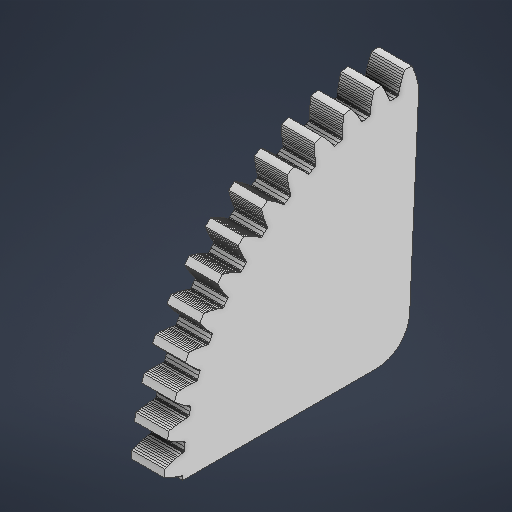
# Autodesk Inventor part: pitch gear v3
Saved by Autodesk Inventor 2026.2 (Build 302298000, 298)
## iProperties
Created: 2026-01-17
Part Number: pitch gear v3
Material: Generic
Document SubType Name: Modeling
Designer: User
Density: 1 g/cm^3
Appearance: Default
Author: User
Autodesk Inventor part; units mm, degrees
(part 1 of 2)
ref_plane "YZ Plane" through (0, 0, 0) normal (1, 0, 0) x (0, 1, 0)
ref_plane "XZ Plane" through (0, 0, 0) normal (0, 1, 0) x (-1, 0, 0)
ref_plane "XY Plane" through (0, 0, 0) normal (0, 0, 1) x (1, 0, 0)
sketch "Sketch1" plane through (0, 0, 0) normal (1, 0, 0) x (0, 1, 0)
  line L0 (51.3338, 5.5368) -> (50.9543, 5.3173)
  line L1 (50.9543, 5.3173) -> (50.5888, 5.1158)
  line L2 (50.5888, 5.1158) -> (50.2381, 4.9321)
  line L3 (50.2381, 4.9321) -> (49.9008, 4.7642)
  line L4 (49.9008, 4.7642) -> (49.5784, 4.6121)
  line L5 (49.5784, 4.6121) -> (49.2732, 4.4759)
  line L6 (49.2732, 4.4759) -> (48.9827, 4.3535)
  line L7 (48.9827, 4.3535) -> (48.455, 4.15)
  line L8 (48.455, 4.15) -> (48.0445, 4.0082)
  line L9 (48.0445, 4.0082) -> (47.95, 3.9663)
  line L10 (47.95, 3.9663) -> (47.8784, 3.9226)
  line L11 (47.8784, 3.9226) -> (47.8295, 3.8782)
  line L12 (47.8295, 3.8782) -> (47.8036, 3.8338)
  line L13 (47.8036, 3.8338) -> (47.7992, 3.812)
  line L14 (47.7992, 3.812) -> (47.812, 3.6369)
  line L15 (47.812, 3.6369) -> (47.8554, 3.0108)
  line L16 (47.8554, 3.0108) -> (47.8909, 2.3842)
  line L17 (47.8909, 2.3842) -> (47.9, 2.2089)
  line L18 (47.9, 2.2089) -> (47.9072, 2.1878)
  line L19 (47.9072, 2.1878) -> (47.9385, 2.1471)
  line L20 (47.9385, 2.1471) -> (47.9925, 2.1091)
  line L21 (47.9925, 2.1091) -> (48.069, 2.0748)
  line L22 (48.069, 2.0748) -> (48.168, 2.045)
  line L23 (48.168, 2.045) -> (48.593, 1.9557)
  line L24 (48.593, 1.9557) -> (49.1421, 1.82)
  line L25 (49.1421, 1.82) -> (49.4456, 1.735)
  line L26 (49.4456, 1.735) -> (49.7655, 1.6381)
  line L27 (49.7655, 1.6381) -> (50.1044, 1.5276)
  line L28 (50.1044, 1.5276) -> (50.4601, 1.4033)
  line L29 (50.4601, 1.4033) -> (50.8311, 1.265)
  line L30 (50.8311, 1.265) -> (51.219, 1.1109)
  line L31 (51.219, 1.1109) -> (51.623, 0.9407)
  line L32 (51.623, 0.9407) -> (51.9942, 0.7753)
  arc A0 (51.9942, -0.7753) -> (51.9942, 0.7753) centre (0, 0) ccw
  line L33 (51.9942, -0.7753) -> (51.623, -0.9407)
  line L34 (51.623, -0.9407) -> (51.219, -1.1109)
  line L35 (51.219, -1.1109) -> (50.8311, -1.265)
  line L36 (50.8311, -1.265) -> (50.4601, -1.4033)
  line L37 (50.4601, -1.4033) -> (50.1044, -1.5276)
  line L38 (50.1044, -1.5276) -> (49.7655, -1.6381)
  line L39 (49.7655, -1.6381) -> (49.4456, -1.735)
  line L40 (49.4456, -1.735) -> (49.1421, -1.82)
  line L41 (49.1421, -1.82) -> (48.593, -1.9557)
  line L42 (48.593, -1.9557) -> (48.168, -2.045)
  line L43 (48.168, -2.045) -> (48.069, -2.0748)
  line L44 (48.069, -2.0748) -> (47.9925, -2.1091)
  line L45 (47.9925, -2.1091) -> (47.9385, -2.1471)
  line L46 (47.9385, -2.1471) -> (47.9072, -2.1878)
  line L47 (47.9072, -2.1878) -> (47.9, -2.2089)
  line L48 (47.9, -2.2089) -> (47.8961, -2.2835)
  line L49 (0, 47.95) -> (0.6276, 47.9461)
  line L50 (0.6276, 47.9461) -> (0.8032, 47.9442)
  line L51 (0.8032, 47.9442) -> (0.8247, 47.95)
  line L52 (0.8247, 47.95) -> (0.8673, 47.9787)
  line L53 (0.8673, 47.9787) -> (0.9086, 48.0302)
  line L54 (0.9086, 48.0302) -> (0.9476, 48.1044)
  line L55 (0.9476, 48.1044) -> (0.9835, 48.2014)
  line L56 (0.9835, 48.2014) -> (1.0993, 48.6199)
  line L57 (1.0993, 48.6199) -> (1.2692, 49.1594)
  line L58 (1.2692, 49.1594) -> (1.3732, 49.457)
  line L59 (1.3732, 49.457) -> (1.49, 49.7701)
  line L60 (1.49, 49.7701) -> (1.6215, 50.1014)
  line L61 (1.6215, 50.1014) -> (1.7678, 50.4486)
  line L62 (1.7678, 50.4486) -> (1.9293, 50.8102)
  line L63 (1.9293, 50.8102) -> (2.1073, 51.1877)
  line L64 (2.1073, 51.1877) -> (2.3026, 51.5802)
  line L65 (2.3026, 51.5802) -> (2.4909, 51.9403)
  arc A1 (4.0386, 51.8429) -> (2.4909, 51.9403) centre (0, 0) ccw
  line L66 (4.0386, 51.8429) -> (4.1802, 51.4621)
  line L67 (4.1802, 51.4621) -> (4.3248, 51.0482)
  line L68 (4.3248, 51.0482) -> (4.4542, 50.6514)
  line L69 (4.4542, 50.6514) -> (4.569, 50.2724)
  line L70 (4.569, 50.2724) -> (4.6707, 49.9096)
  line L71 (4.6707, 49.9096) -> (4.7596, 49.5644)
  line L72 (4.7596, 49.5644) -> (4.8363, 49.2391)
  line L73 (4.8363, 49.2391) -> (4.9021, 48.9308)
  line L74 (4.9021, 48.9308) -> (5.003, 48.3743)
  line L75 (5.003, 48.3743) -> (5.0655, 47.9445)
  line L76 (5.0655, 47.9445) -> (5.0889, 47.8439)
  line L77 (5.0889, 47.8439) -> (5.1184, 47.7653)
  line L78 (5.1184, 47.7653) -> (5.1529, 47.7091)
  line L79 (5.1529, 47.7091) -> (5.1916, 47.6753)
  line L80 (5.1916, 47.6753) -> (5.2122, 47.6668)
  line L81 (5.2122, 47.6668) -> (5.3866, 47.6467)
  line L82 (5.3866, 47.6467) -> (6.0097, 47.5719)
  line L83 (6.0097, 47.5719) -> (6.6319, 47.4893)
  line L84 (6.6319, 47.4893) -> (6.8058, 47.4655)
  line L85 (6.8058, 47.4655) -> (6.8279, 47.4685)
  line L86 (6.8279, 47.4685) -> (6.8737, 47.4917)
  line L87 (6.8737, 47.4917) -> (6.9212, 47.5376)
  line L88 (6.9212, 47.5376) -> (6.9692, 47.6063)
  line L89 (6.9692, 47.6063) -> (7.017, 47.698)
  line L90 (7.017, 47.698) -> (7.1844, 48.0988)
  line L91 (7.1844, 48.0988) -> (7.4205, 48.6127)
  line L92 (7.4205, 48.6127) -> (7.5609, 48.8949)
  line L93 (7.5609, 48.8949) -> (7.7161, 49.1909)
  line L94 (7.7161, 49.1909) -> (7.8881, 49.5031)
  line L95 (7.8881, 49.5031) -> (8.0768, 49.8293)
  line L96 (8.0768, 49.8293) -> (8.2822, 50.1678)
  line L97 (8.2822, 50.1678) -> (8.5062, 50.5199)
  line L98 (8.5062, 50.5199) -> (8.7492, 50.8849)
  line L99 (8.7492, 50.8849) -> (8.9811, 51.2185)
  arc A2 (10.5044, 50.928) -> (8.9811, 51.2185) centre (0, 0) ccw
  line L100 (10.5044, 50.928) -> (10.5972, 50.5323)
  line L101 (10.5972, 50.5323) -> (10.6888, 50.1036)
  line L102 (10.6888, 50.1036) -> (10.7673, 49.6937)
  line L103 (10.7673, 49.6937) -> (10.8338, 49.3033)
  line L104 (10.8338, 49.3033) -> (10.8892, 48.9306)
  line L105 (10.8892, 48.9306) -> (10.9342, 48.5771)
  line L106 (10.9342, 48.5771) -> (10.9694, 48.2447)
  line L107 (10.9694, 48.2447) -> (10.9961, 47.9306)
  line L108 (10.9961, 47.9306) -> (11.0265, 47.3658)
  line L109 (11.0265, 47.3658) -> (11.0346, 46.9316)
  line L110 (11.0346, 46.9316) -> (11.0452, 46.8288)
  line L111 (11.0452, 46.8288) -> (11.0646, 46.7472)
  line L112 (11.0646, 46.7472) -> (11.0918, 46.687)
  line L113 (11.0918, 46.687) -> (11.1259, 46.6486)
  line L114 (11.1259, 46.6486) -> (11.1453, 46.6377)
  line L115 (11.1453, 46.6377) -> (11.3158, 46.5958)
  line L116 (11.3158, 46.5958) -> (11.9247, 46.4436)
  line L117 (11.9247, 46.4436) -> (12.5316, 46.2837)
  line L118 (12.5316, 46.2837) -> (12.7012, 46.2382)
  line L119 (12.7012, 46.2382) -> (12.7234, 46.2385)
  line L120 (12.7234, 46.2385) -> (12.7718, 46.2557)
  line L121 (12.7718, 46.2557) -> (12.8246, 46.2953)
  line L122 (12.8246, 46.2953) -> (12.8809, 46.3575)
  line L123 (12.8809, 46.3575) -> (12.9398, 46.4424)
  line L124 (12.9398, 46.4424) -> (13.1561, 46.819)
  line L125 (13.1561, 46.819) -> (13.4548, 47.2993)
  line L126 (13.4548, 47.2993) -> (13.6295, 47.5617)
  line L127 (13.6295, 47.5617) -> (13.8205, 47.836)
  line L128 (13.8205, 47.836) -> (14.0303, 48.1242)
  line L129 (14.0303, 48.1242) -> (14.2584, 48.4241)
  line L130 (14.2584, 48.4241) -> (14.5046, 48.7341)
  line L131 (14.5046, 48.7341) -> (14.771, 49.0554)
  line L132 (14.771, 49.0554) -> (15.0578, 49.3871)
  line L133 (15.0578, 49.3871) -> (15.3297, 49.689)
  arc A3 (16.8045, 49.2098) -> (15.3297, 49.689) centre (0, 0) ccw
  line L134 (16.8045, 49.2098) -> (16.847, 48.8057)
  line L135 (16.847, 48.8057) -> (16.8841, 48.3688)
  line L136 (16.8841, 48.3688) -> (16.9107, 47.9523)
  line L137 (16.9107, 47.9523) -> (16.9277, 47.5567)
  line L138 (16.9277, 47.5567) -> (16.9359, 47.18)
  line L139 (16.9359, 47.18) -> (16.9363, 46.8236)
  line L140 (16.9363, 46.8236) -> (16.9296, 46.4894)
  line L141 (16.9296, 46.4894) -> (16.9167, 46.1745)
  line L142 (16.9167, 46.1745) -> (16.876, 45.6104)
  line L143 (16.876, 45.6104) -> (16.8297, 45.1785)
  line L144 (16.8297, 45.1785) -> (16.8273, 45.0752)
  line L145 (16.8273, 45.0752) -> (16.8363, 44.9918)
  line L146 (16.8363, 44.9918) -> (16.8558, 44.9287)
  line L147 (16.8558, 44.9287) -> (16.8848, 44.8864)
  line L148 (16.8848, 44.8864) -> (16.9027, 44.8731)
  line L149 (16.9027, 44.8731) -> (17.0666, 44.8102)
  line L150 (17.0666, 44.8102) -> (17.6516, 44.5828)
  line L151 (17.6516, 44.5828) -> (18.2337, 44.3481)
  line L152 (18.2337, 44.3481) -> (18.3962, 44.2817)
  line L153 (18.3962, 44.2817) -> (18.4183, 44.2792)
  line L154 (18.4183, 44.2792) -> (18.4685, 44.2902)
  line L155 (18.4685, 44.2902) -> (18.5258, 44.3229)
  line L156 (18.5258, 44.3229) -> (18.5895, 44.3775)
  line L157 (18.5895, 44.3775) -> (18.6585, 44.4544)
  line L158 (18.6585, 44.4544) -> (18.9203, 44.801)
  line L159 (18.9203, 44.801) -> (19.2769, 45.24)
  line L160 (19.2769, 45.24) -> (19.4831, 45.4785)
  line L161 (19.4831, 45.4785) -> (19.7069, 45.7266)
  line L162 (19.7069, 45.7266) -> (19.9512, 45.9862)
  line L163 (19.9512, 45.9862) -> (20.2151, 46.2552)
  line L164 (20.2151, 46.2552) -> (20.4983, 46.5319)
  line L165 (20.4983, 46.5319) -> (20.8028, 46.8173)
  line L166 (20.8028, 46.8173) -> (21.1289, 47.1104)
  line L167 (21.1289, 47.1104) -> (21.4365, 47.3759)
  arc A4 (22.8396, 46.7156) -> (21.4365, 47.3759) centre (0, 0) ccw
  line L168 (22.8396, 46.7156) -> (22.8311, 46.3094)
  line L169 (22.8311, 46.3094) -> (22.8132, 45.8713)
  line L170 (22.8132, 45.8713) -> (22.7874, 45.4547)
  line L171 (22.7874, 45.4547) -> (22.7546, 45.0601)
  line L172 (22.7546, 45.0601) -> (22.7156, 44.6854)
  line L173 (22.7156, 44.6854) -> (22.6713, 44.3317)
  line L174 (22.6713, 44.3317) -> (22.6228, 44.001)
  line L175 (22.6228, 44.001) -> (22.5705, 43.6902)
  line L176 (22.5705, 43.6902) -> (22.4595, 43.1356)
  line L177 (22.4595, 43.1356) -> (22.3593, 42.713)
  line L178 (22.3593, 42.713) -> (22.3441, 42.6107)
  line L179 (22.3441, 42.6107) -> (22.3425, 42.5269)
  line L180 (22.3425, 42.5269) -> (22.3539, 42.4618)
  line L181 (22.3539, 42.4618) -> (22.3774, 42.4162)
  line L182 (22.3774, 42.4162) -> (22.3935, 42.4008)
  line L183 (22.3935, 42.4008) -> (22.5482, 42.3178)
  line L184 (22.5482, 42.3178) -> (23.1001, 42.0189)
  line L185 (23.1001, 42.0189) -> (23.6482, 41.7131)
  line L186 (23.6482, 41.7131) -> (23.8011, 41.6269)
  line L187 (23.8011, 41.6269) -> (23.8227, 41.6216)
  line L188 (23.8227, 41.6216) -> (23.8739, 41.6262)
  line L189 (23.8739, 41.6262) -> (23.9349, 41.6515)
  line L190 (23.9349, 41.6515) -> (24.0049, 41.6977)
  line L191 (24.0049, 41.6977) -> (24.083, 41.7654)
  line L192 (24.083, 41.7654) -> (24.3862, 42.0763)
  line L193 (24.3862, 42.0763) -> (24.7949, 42.4673)
  line L194 (24.7949, 42.4673) -> (25.0294, 42.678)
  line L195 (25.0294, 42.678) -> (25.2826, 42.8961)
  line L196 (25.2826, 42.8961) -> (25.5575, 43.1231)
  line L197 (25.5575, 43.1231) -> (25.853, 43.3568)
  line L198 (25.853, 43.3568) -> (26.1686, 43.5959)
  line L199 (26.1686, 43.5959) -> (26.5065, 43.8409)
  line L200 (26.5065, 43.8409) -> (26.8668, 44.0908)
  line L201 (26.8668, 44.0908) -> (27.2052, 44.3156)
  arc A5 (28.5145, 43.4847) -> (27.2052, 44.3156) centre (0, 0) ccw
  line L202 (28.5145, 43.4847) -> (28.4552, 43.0827)
  line L203 (28.4552, 43.0827) -> (28.3825, 42.6503)
  line L204 (28.3825, 42.6503) -> (28.3047, 42.2403)
  line L205 (28.3047, 42.2403) -> (28.2227, 41.8529)
  line L206 (28.2227, 41.8529) -> (28.1371, 41.486)
  line L207 (28.1371, 41.486) -> (28.0488, 41.1407)
  line L208 (28.0488, 41.1407) -> (27.9592, 40.8187)
  line L209 (27.9592, 40.8187) -> (27.8684, 40.5168)
  line L210 (27.8684, 40.5168) -> (27.6887, 39.9805)
  line L211 (27.6887, 39.9805) -> (27.5364, 39.5738)
  line L212 (27.5364, 39.5738) -> (27.5084, 39.4743)
  line L213 (27.5084, 39.4743) -> (27.4964, 39.3913)
  line L214 (27.4964, 39.3913) -> (27.4995, 39.3253)
  line L215 (27.4995, 39.3253) -> (27.5171, 39.2771)
  line L216 (27.5171, 39.2771) -> (27.5311, 39.2598)
  line L217 (27.5311, 39.2598) -> (27.6742, 39.1581)
  line L218 (27.6742, 39.1581) -> (28.1843, 38.7924)
  line L219 (28.1843, 38.7924) -> (28.6898, 38.4203)
  line L220 (28.6898, 38.4203) -> (28.8307, 38.3156)
  line L221 (28.8307, 38.3156) -> (28.8515, 38.3076)
  line L222 (28.8515, 38.3076) -> (28.9028, 38.3058)
  line L223 (28.9028, 38.3058) -> (28.9665, 38.3232)
  line L224 (28.9665, 38.3232) -> (29.0417, 38.3603)
  line L225 (29.0417, 38.3603) -> (29.1277, 38.4176)
  line L226 (29.1277, 38.4176) -> (29.4675, 38.6882)
  line L227 (29.4675, 38.6882) -> (29.922, 39.0248)
  line L228 (29.922, 39.0248) -> (30.181, 39.2044)
  line L229 (30.181, 39.2044) -> (30.4596, 39.3891)
  line L230 (30.4596, 39.3891) -> (30.7607, 39.5798)
  line L231 (30.7607, 39.5798) -> (31.0832, 39.7747)
  line L232 (31.0832, 39.7747) -> (31.4263, 39.9723)
  line L233 (31.4263, 39.9723) -> (31.7922, 40.173)
  line L234 (31.7922, 40.173) -> (32.1809, 40.3758)
  line L235 (32.1809, 40.3758) -> (32.5449, 40.5565)
  arc A6 (33.7398, 39.568) -> (32.5449, 40.5565) centre (0, 0) ccw
  line L236 (33.7398, 39.568) -> (33.6305, 39.1766)
  line L237 (33.6305, 39.1766) -> (33.5042, 38.7568)
  line L238 (33.5042, 38.7568) -> (33.3756, 38.3597)
  line L239 (33.3756, 38.3597) -> (33.2458, 37.9857)
  line L240 (33.2458, 37.9857) -> (33.1148, 37.6324)
  line L241 (33.1148, 37.6324) -> (32.9839, 37.3008)
  line L242 (32.9839, 37.3008) -> (32.8546, 36.9926)
  line L243 (32.8546, 36.9926) -> (32.7267, 36.7045)
  line L244 (32.7267, 36.7045) -> (32.4812, 36.1949)
  line L245 (32.4812, 36.1949) -> (32.2791, 35.8105)
  line L246 (32.2791, 35.8105) -> (32.239, 35.7153)
  line L247 (32.239, 35.7153) -> (32.2166, 35.6344)
  line L248 (32.2166, 35.6344) -> (32.2115, 35.5686)
  line L249 (32.2115, 35.5686) -> (32.2229, 35.5186)
  line L250 (32.2229, 35.5186) -> (32.2346, 35.4996)
  line L251 (32.2346, 35.4996) -> (32.3638, 35.3808)
  line L252 (32.3638, 35.3808) -> (32.824, 34.954)
  line L253 (32.824, 34.954) -> (33.2789, 34.5215)
  line L254 (33.2789, 34.5215) -> (33.4056, 34.4)
  line L255 (33.4056, 34.4) -> (33.4252, 34.3895)
  line L256 (33.4252, 34.3895) -> (33.4759, 34.3813)
  line L257 (33.4759, 34.3813) -> (33.5412, 34.3905)
  line L258 (33.5412, 34.3905) -> (33.6205, 34.4179)
  line L259 (33.6205, 34.4179) -> (33.713, 34.464)
  line L260 (33.713, 34.464) -> (34.084, 34.6898)
  line L261 (34.084, 34.6898) -> (34.5771, 34.9668)
  line L262 (34.5771, 34.9668) -> (34.8566, 35.1126)
  line L263 (34.8566, 35.1126) -> (35.1561, 35.2609)
  line L264 (35.1561, 35.2609) -> (35.4788, 35.4124)
  line L265 (35.4788, 35.4124) -> (35.8232, 35.5653)
  line L266 (35.8232, 35.5653) -> (36.1883, 35.7184)
  line L267 (36.1883, 35.7184) -> (36.5765, 35.8717)
  line L268 (36.5765, 35.8717) -> (36.9876, 36.0241)
  line L269 (36.9876, 36.0241) -> (37.3714, 36.1577)
  arc A7 (38.4329, 35.0273) -> (37.3714, 36.1577) centre (0, 0) ccw
  line L270 (38.4329, 35.0273) -> (38.2755, 34.6527)
  line L271 (38.2755, 34.6527) -> (38.0975, 34.252)
  line L272 (38.0975, 34.252) -> (37.9202, 33.8742)
  line L273 (37.9202, 33.8742) -> (37.7445, 33.5193)
  line L274 (37.7445, 33.5193) -> (37.5702, 33.1852)
  line L275 (37.5702, 33.1852) -> (37.3988, 32.8727)
  line L276 (37.3988, 32.8727) -> (37.232, 32.5831)
  line L277 (37.232, 32.5831) -> (37.069, 32.3133)
  line L278 (37.069, 32.3133) -> (36.7615, 31.8386)
  line L279 (36.7615, 31.8386) -> (36.5129, 31.4825)
  line L280 (36.5129, 31.4825) -> (36.4611, 31.3931)
  line L281 (36.4611, 31.3931) -> (36.4288, 31.3156)
  line L282 (36.4288, 31.3156) -> (36.4154, 31.251)
  line L283 (36.4154, 31.251) -> (36.4205, 31.1999)
  line L284 (36.4205, 31.1999) -> (36.4297, 31.1796)
  line L285 (36.4297, 31.1796) -> (36.543, 31.0456)
  line L286 (36.543, 31.0456) -> (36.9461, 30.5645)
  line L287 (36.9461, 30.5645) -> (37.3431, 30.0784)
  line L288 (37.3431, 30.0784) -> (37.4536, 29.942)
  line L289 (37.4536, 29.942) -> (37.4718, 29.9291)
  line L290 (37.4718, 29.9291) -> (37.521, 29.9145)
  line L291 (37.521, 29.9145) -> (37.587, 29.9155)
  line L292 (37.587, 29.9155) -> (37.6691, 29.9328)
  line L293 (37.6691, 29.9328) -> (37.7667, 29.9669)
  line L294 (37.7667, 29.9669) -> (38.163, 30.1444)
  line L295 (38.163, 30.1444) -> (38.687, 30.3574)
  line L296 (38.687, 30.3574) -> (38.9826, 30.467)
  line L297 (38.9826, 30.467) -> (39.2983, 30.5766)
  line L298 (39.2983, 30.5766) -> (39.6374, 30.6865)
  line L299 (39.6374, 30.6865) -> (39.9982, 30.795)
  line L300 (39.9982, 30.795) -> (40.3797, 30.9011)
  line L301 (40.3797, 30.9011) -> (40.784, 31.0045)
  line L302 (40.784, 31.0045) -> (41.211, 31.1042)
  line L303 (41.211, 31.1042) -> (41.6085, 31.1887)
  arc A8 (42.5199, 29.9342) -> (41.6085, 31.1887) centre (0, 0) ccw
  line L304 (42.5199, 29.9342) -> (42.3168, 29.5822)
  line L305 (42.3168, 29.5822) -> (42.09, 29.207)
  line L306 (42.09, 29.207) -> (41.8667, 28.8544)
  line L307 (41.8667, 28.8544) -> (41.6479, 28.5244)
  line L308 (41.6479, 28.5244) -> (41.4332, 28.2148)
  line L309 (41.4332, 28.2148) -> (41.224, 27.9262)
  line L310 (41.224, 27.9262) -> (41.0221, 27.6598)
  line L311 (41.0221, 27.6598) -> (40.8266, 27.4126)
  line L312 (40.8266, 27.4126) -> (40.4621, 26.9801)
  line L313 (40.4621, 26.9801) -> (40.1708, 26.658)
  line L314 (40.1708, 26.658) -> (40.1081, 26.5757)
  line L315 (40.1081, 26.5757) -> (40.0664, 26.503)
  line L316 (40.0664, 26.503) -> (40.045, 26.4405)
  line L317 (40.045, 26.4405) -> (40.0436, 26.3892)
  line L318 (40.0436, 26.3892) -> (40.0503, 26.3679)
  line L319 (40.0503, 26.3679) -> (40.1459, 26.2207)
  line L320 (40.1459, 26.2207) -> (40.4855, 25.6929)
  line L321 (40.4855, 25.6929) -> (40.8185, 25.1609)
  line L322 (40.8185, 25.1609) -> (40.911, 25.0117)
  line L323 (40.911, 25.0117) -> (40.9274, 24.9966)
  line L324 (40.9274, 24.9966) -> (40.9744, 24.976)
  line L325 (40.9744, 24.976) -> (41.04, 24.9687)
  line L326 (41.04, 24.9687) -> (41.1237, 24.9755)
  line L327 (41.1237, 24.9755) -> (41.2247, 24.9972)
  line L328 (41.2247, 24.9972) -> (41.6402, 25.1237)
  line L329 (41.6402, 25.1237) -> (42.1867, 25.2693)
  line L330 (42.1867, 25.2693) -> (42.4937, 25.341)
  line L331 (42.4937, 25.341) -> (42.8207, 25.4102)
  line L332 (42.8207, 25.4102) -> (43.1709, 25.4766)
  line L333 (43.1709, 25.4766) -> (43.5425, 25.5391)
  line L334 (43.5425, 25.5391) -> (43.9342, 25.5966)
  line L335 (43.9342, 25.5966) -> (44.3483, 25.6485)
  line L336 (44.3483, 25.6485) -> (44.7844, 25.6939)
  line L337 (44.7844, 25.6939) -> (45.1894, 25.7278)
  arc A9 (45.9364, 24.369) -> (45.1894, 25.7278) centre (0, 0) ccw
  line L338 (45.9364, 24.369) -> (45.6907, 24.0453)
  line L339 (45.6907, 24.0453) -> (45.4187, 23.7014)
  line L340 (45.4187, 23.7014) -> (45.153, 23.3796)
  line L341 (45.153, 23.3796) -> (44.8946, 23.0796)
  line L342 (44.8946, 23.0796) -> (44.6427, 22.7993)
  line L343 (44.6427, 22.7993) -> (44.399, 22.5393)
  line L344 (44.399, 22.5393) -> (44.1654, 22.3002)
  line L345 (44.1654, 22.3002) -> (43.9404, 22.0795)
  line L346 (43.9404, 22.0795) -> (43.5245, 21.6961)
  line L347 (43.5245, 21.6961) -> (43.1951, 21.413)
  line L348 (43.1951, 21.413) -> (43.1227, 21.3393)
  line L349 (43.1227, 21.3393) -> (43.0722, 21.2723)
  line L350 (43.0722, 21.2723) -> (43.0431, 21.213)
  line L351 (43.0431, 21.213) -> (43.0353, 21.1623)
  line L352 (43.0353, 21.1623) -> (43.0393, 21.1404)
  line L353 (43.0393, 21.1404) -> (43.1157, 20.9823)
  line L354 (43.1157, 20.9823) -> (43.3865, 20.4161)
  line L355 (43.3865, 20.4161) -> (43.6501, 19.8465)
  line L356 (43.6501, 19.8465) -> (43.7232, 19.6869)
  line L357 (43.7232, 19.6869) -> (43.7376, 19.6699)
  line L358 (43.7376, 19.6699) -> (43.7817, 19.6436)
  line L359 (43.7817, 19.6436) -> (43.8458, 19.6282)
  line L360 (43.8458, 19.6282) -> (43.9297, 19.6244)
  line L361 (43.9297, 19.6244) -> (44.0326, 19.6332)
  line L362 (44.0326, 19.6332) -> (44.4607, 19.7066)
  line L363 (44.4607, 19.7066) -> (45.0212, 19.7826)
  line L364 (45.0212, 19.7826) -> (45.3347, 19.8153)
  line L365 (45.3347, 19.8153) -> (45.6678, 19.8429)
  line L366 (45.6678, 19.8429) -> (46.0235, 19.865)
  line L367 (46.0235, 19.865) -> (46.4, 19.8804)
  line L368 (46.4, 19.8804) -> (46.7959, 19.8883)
  line L369 (46.7959, 19.8883) -> (47.2132, 19.8879)
  line L370 (47.2132, 19.8879) -> (47.6516, 19.8783)
  line L371 (47.6516, 19.8783) -> (48.0576, 19.8612)
  arc A10 (48.6284, 18.4194) -> (48.0576, 19.8612) centre (0, 0) ccw
  line L372 (48.6284, 18.4194) -> (48.3441, 18.1291)
  line L373 (48.3441, 18.1291) -> (48.0312, 17.822)
  line L374 (48.0312, 17.822) -> (47.7272, 17.536)
  line L375 (47.7272, 17.536) -> (47.4332, 17.2708)
  line L376 (47.4332, 17.2708) -> (47.1482, 17.0243)
  line L377 (47.1482, 17.0243) -> (46.8738, 16.7969)
  line L378 (46.8738, 16.7969) -> (46.6121, 16.589)
  line L379 (46.6121, 16.589) -> (46.3612, 16.3982)
  line L380 (46.3612, 16.3982) -> (45.9006, 16.0699)
  line L381 (45.9006, 16.0699) -> (45.5383, 15.8304)
  line L382 (45.5383, 15.8304) -> (45.4572, 15.7663)
  line L383 (45.4572, 15.7663) -> (45.3987, 15.7062)
  line L384 (45.3987, 15.7062) -> (45.3624, 15.651)
  line L385 (45.3624, 15.651) -> (45.3483, 15.6017)
  line L386 (45.3483, 15.6017) -> (45.3495, 15.5794)
  line L387 (45.3495, 15.5794) -> (45.4055, 15.4131)
  line L388 (45.4055, 15.4131) -> (45.6032, 14.8174)
  line L389 (45.6032, 14.8174) -> (45.7934, 14.2192)
  line L390 (45.7934, 14.2192) -> (45.8459, 14.0517)
  line L391 (45.8459, 14.0517) -> (45.858, 14.0331)
  line L392 (45.858, 14.0331) -> (45.8984, 14.0014)
  line L393 (45.8984, 14.0014) -> (45.9602, 13.9781)
  line L394 (45.9602, 13.9781) -> (46.0429, 13.9638)
  line L395 (46.0429, 13.9638) -> (46.1461, 13.9597)
  line L396 (46.1461, 13.9597) -> (46.58, 13.9788)
  line L397 (46.58, 13.9788) -> (47.1456, 13.984)
  line L398 (47.1456, 13.984) -> (47.4607, 13.9771)
  line L399 (47.4607, 13.9771) -> (47.7946, 13.9628)
  line L400 (47.7946, 13.9628) -> (48.1504, 13.9401)
  line L401 (48.1504, 13.9401) -> (48.5258, 13.9082)
  line L402 (48.5258, 13.9082) -> (48.9196, 13.8664)
  line L403 (48.9196, 13.8664) -> (49.3336, 13.8137)
  line L404 (49.3336, 13.8137) -> (49.7672, 13.7492)
  line L405 (49.7672, 13.7492) -> (50.1679, 13.6814)
  arc A11 (50.5535, 12.1794) -> (50.1679, 13.6814) centre (0, 0) ccw
  line L406 (50.5535, 12.1794) -> (50.2351, 11.927)
  line L407 (50.2351, 11.927) -> (49.8861, 11.6616)
  line L408 (49.8861, 11.6616) -> (49.5487, 11.416)
  line L409 (49.5487, 11.416) -> (49.2238, 11.1897)
  line L410 (49.2238, 11.1897) -> (48.9102, 10.9808)
  line L411 (48.9102, 10.9808) -> (48.6094, 10.7896)
  line L412 (48.6094, 10.7896) -> (48.3237, 10.6162)
  line L413 (48.3237, 10.6162) -> (48.0508, 10.4583)
  line L414 (48.0508, 10.4583) -> (47.5527, 10.1903)
  line L415 (47.5527, 10.1903) -> (47.1633, 9.9981)
  line L416 (47.1633, 9.9981) -> (47.0748, 9.9447)
  line L417 (47.0748, 9.9447) -> (47.0092, 9.8924)
  line L418 (47.0092, 9.8924) -> (46.9663, 9.8422)
  line L419 (46.9663, 9.8422) -> (46.9461, 9.795)
  line L420 (46.9461, 9.795) -> (46.9445, 9.7728)
  line L421 (46.9445, 9.7728) -> (46.9792, 9.6007)
  line L422 (46.9792, 9.6007) -> (47.1007, 8.9849)
  line L423 (47.1007, 8.9849) -> (47.2144, 8.3677)
  line L424 (47.2144, 8.3677) -> (47.2455, 8.1949)
  line L425 (47.2455, 8.1949) -> (47.2552, 8.1749)
  line L426 (47.2552, 8.1749) -> (47.2914, 8.1384)
  line L427 (47.2914, 8.1384) -> (47.3497, 8.1075)
  line L428 (47.3497, 8.1075) -> (47.4299, 8.083)
  line L429 (47.4299, 8.083) -> (47.5319, 8.0659)
  line L430 (47.5319, 8.0659) -> (47.9647, 8.0306)
  line L431 (47.9647, 8.0306) -> (48.5265, 7.9648)
  line L432 (48.5265, 7.9648) -> (48.8383, 7.9185)
  line L433 (48.8383, 7.9185) -> (49.1678, 7.8624)
  line L434 (49.1678, 7.8624) -> (49.5178, 7.7953)
  line L435 (49.5178, 7.7953) -> (49.8863, 7.7166)
  line L436 (49.8863, 7.7166) -> (50.2717, 7.6258)
  line L437 (50.2717, 7.6258) -> (50.6759, 7.5216)
  line L438 (50.6759, 7.5216) -> (51.098, 7.4033)
  line L439 (51.098, 7.4033) -> (51.487, 7.2858)
  arc A12 (51.6814, 5.7474) -> (51.487, 7.2858) centre (0, 0) ccw
  line L440 (51.6814, 5.7474) -> (51.3338, 5.5368)
  line L441 (51.3338, 5.5368) -> (50.9543, 5.3173)
  line L442 (50.9543, 5.3173) -> (50.5888, 5.1158)
  line L443 (50.5888, 5.1158) -> (50.2381, 4.9321)
  line L444 (50.2381, 4.9321) -> (49.9008, 4.7642)
  line L445 (49.9008, 4.7642) -> (49.5784, 4.6121)
  line L446 (49.5784, 4.6121) -> (49.2732, 4.4759)
  line L447 (49.2732, 4.4759) -> (48.9827, 4.3535)
  line L448 (48.9827, 4.3535) -> (48.455, 4.15)
  line L449 (48.455, 4.15) -> (48.0445, 4.0082)
  line L450 (48.0445, 4.0082) -> (47.95, 3.9663)
  line L451 (47.95, 3.9663) -> (47.8784, 3.9226)
  line L452 (47.8784, 3.9226) -> (47.8295, 3.8782)
  line L453 (47.8295, 3.8782) -> (47.8036, 3.8338)
  line L454 (47.8036, 3.8338) -> (47.7992, 3.812)
  line L455 (47.7992, 3.812) -> (47.812, 3.6369)
  line L456 (47.812, 3.6369) -> (47.8554, 3.0108)
  line L457 (47.8554, 3.0108) -> (47.8909, 2.3842)
  line L458 (47.8909, 2.3842) -> (47.9, 2.2089)
  line L459 (47.9, 2.2089) -> (47.9072, 2.1878)
  line L460 (47.9072, 2.1878) -> (47.9385, 2.1471)
  line L461 (47.9385, 2.1471) -> (47.9925, 2.1091)
  line L462 (47.9925, 2.1091) -> (48.069, 2.0748)
  line L463 (48.069, 2.0748) -> (48.168, 2.045)
  line L464 (48.168, 2.045) -> (48.593, 1.9557)
  line L465 (48.593, 1.9557) -> (49.1421, 1.82)
  line L466 (49.1421, 1.82) -> (49.4456, 1.735)
  line L467 (49.4456, 1.735) -> (49.7655, 1.6381)
  line L468 (49.7655, 1.6381) -> (50.1044, 1.5276)
  line L469 (50.1044, 1.5276) -> (50.4601, 1.4033)
  line L470 (50.4601, 1.4033) -> (50.8311, 1.265)
  line L471 (50.8311, 1.265) -> (51.219, 1.1109)
  line L472 (51.219, 1.1109) -> (51.623, 0.9407)
  line L473 (51.623, 0.9407) -> (51.9942, 0.7753)
  arc A13 (51.9942, -0.7753) -> (51.9942, 0.7753) centre (0, 0) ccw
  line L474 (51.9942, -0.7753) -> (51.623, -0.9407)
  line L475 (51.623, -0.9407) -> (51.219, -1.1109)
  line L476 (51.219, -1.1109) -> (50.8311, -1.265)
  line L477 (50.8311, -1.265) -> (50.4601, -1.4033)
  line L478 (50.4601, -1.4033) -> (50.1044, -1.5276)
  line L479 (50.1044, -1.5276) -> (49.7655, -1.6381)
  line L480 (49.7655, -1.6381) -> (49.4456, -1.735)
  line L481 (49.4456, -1.735) -> (49.1421, -1.82)
  line L482 (49.1421, -1.82) -> (48.593, -1.9557)
  line L483 (48.593, -1.9557) -> (48.168, -2.045)
  line L484 (48.168, -2.045) -> (48.069, -2.0748)
  line L485 (48.069, -2.0748) -> (47.9925, -2.1091)
  line L486 (47.9925, -2.1091) -> (47.9385, -2.1471)
  line L487 (47.9385, -2.1471) -> (47.9072, -2.1878)
  line L488 (47.9072, -2.1878) -> (47.9, -2.2089)
  line L489 (47.9, -2.2089) -> (47.8961, -2.2835)
  line L490 (0, 47.95) -> (0.6276, 47.9461)
  line L491 (0.6276, 47.9461) -> (0.8032, 47.9442)
  line L492 (0.8032, 47.9442) -> (0.8247, 47.95)
  line L493 (0.8247, 47.95) -> (0.8673, 47.9787)
  line L494 (0.8673, 47.9787) -> (0.9086, 48.0302)
  line L495 (0.9086, 48.0302) -> (0.9476, 48.1044)
  line L496 (0.9476, 48.1044) -> (0.9835, 48.2014)
  line L497 (0.9835, 48.2014) -> (1.0993, 48.6199)
  line L498 (1.0993, 48.6199) -> (1.2692, 49.1594)
  line L499 (1.2692, 49.1594) -> (1.3732, 49.457)
  line L500 (1.3732, 49.457) -> (1.49, 49.7701)
  line L501 (1.49, 49.7701) -> (1.6215, 50.1014)
  line L502 (1.6215, 50.1014) -> (1.7678, 50.4486)
  line L503 (1.7678, 50.4486) -> (1.9293, 50.8102)
  line L504 (1.9293, 50.8102) -> (2.1073, 51.1877)
  line L505 (2.1073, 51.1877) -> (2.3026, 51.5802)
  line L506 (2.3026, 51.5802) -> (2.4909, 51.9403)
  arc A14 (4.0386, 51.8429) -> (2.4909, 51.9403) centre (0, 0) ccw
  line L507 (4.0386, 51.8429) -> (4.1802, 51.4621)
  line L508 (4.1802, 51.4621) -> (4.3248, 51.0482)
  line L509 (4.3248, 51.0482) -> (4.4542, 50.6514)
  line L510 (4.4542, 50.6514) -> (4.569, 50.2724)
  line L511 (4.569, 50.2724) -> (4.6707, 49.9096)
  line L512 (4.6707, 49.9096) -> (4.7596, 49.5644)
  line L513 (4.7596, 49.5644) -> (4.8363, 49.2391)
  line L514 (4.8363, 49.2391) -> (4.9021, 48.9308)
  line L515 (4.9021, 48.9308) -> (5.003, 48.3743)
  line L516 (5.003, 48.3743) -> (5.0655, 47.9445)
  line L517 (5.0655, 47.9445) -> (5.0889, 47.8439)
  line L518 (5.0889, 47.8439) -> (5.1184, 47.7653)
  line L519 (5.1184, 47.7653) -> (5.1529, 47.7091)
  line L520 (5.1529, 47.7091) -> (5.1916, 47.6753)
  line L521 (5.1916, 47.6753) -> (5.2122, 47.6668)
  line L522 (5.2122, 47.6668) -> (5.3866, 47.6467)
  line L523 (5.3866, 47.6467) -> (6.0097, 47.5719)
  line L524 (6.0097, 47.5719) -> (6.6319, 47.4893)
  line L525 (6.6319, 47.4893) -> (6.8058, 47.4655)
  line L526 (6.8058, 47.4655) -> (6.8279, 47.4685)
  line L527 (6.8279, 47.4685) -> (6.8737, 47.4917)
  line L528 (6.8737, 47.4917) -> (6.9212, 47.5376)
  line L529 (6.9212, 47.5376) -> (6.9692, 47.6063)
  line L530 (6.9692, 47.6063) -> (7.017, 47.698)
  line L531 (7.017, 47.698) -> (7.1844, 48.0988)
  line L532 (7.1844, 48.0988) -> (7.4205, 48.6127)
  line L533 (7.4205, 48.6127) -> (7.5609, 48.8949)
  line L534 (7.5609, 48.8949) -> (7.7161, 49.1909)
  line L535 (7.7161, 49.1909) -> (7.8881, 49.5031)
  line L536 (7.8881, 49.5031) -> (8.0768, 49.8293)
  line L537 (8.0768, 49.8293) -> (8.2822, 50.1678)
  line L538 (8.2822, 50.1678) -> (8.5062, 50.5199)
  line L539 (8.5062, 50.5199) -> (8.7492, 50.8849)
  line L540 (8.7492, 50.8849) -> (8.9811, 51.2185)
  arc A15 (10.5044, 50.928) -> (8.9811, 51.2185) centre (0, 0) ccw
  line L541 (10.5044, 50.928) -> (10.5972, 50.5323)
  line L542 (10.5972, 50.5323) -> (10.6888, 50.1036)
  line L543 (10.6888, 50.1036) -> (10.7673, 49.6937)
  line L544 (10.7673, 49.6937) -> (10.8338, 49.3033)
  line L545 (10.8338, 49.3033) -> (10.8892, 48.9306)
  line L546 (10.8892, 48.9306) -> (10.9342, 48.5771)
  line L547 (10.9342, 48.5771) -> (10.9694, 48.2447)
  line L548 (10.9694, 48.2447) -> (10.9961, 47.9306)
  line L549 (10.9961, 47.9306) -> (11.0265, 47.3658)
  line L550 (11.0265, 47.3658) -> (11.0346, 46.9316)
  line L551 (11.0346, 46.9316) -> (11.0452, 46.8288)
  line L552 (11.0452, 46.8288) -> (11.0646, 46.7472)
  line L553 (11.0646, 46.7472) -> (11.0918, 46.687)
  line L554 (11.0918, 46.687) -> (11.1259, 46.6486)
  line L555 (11.1259, 46.6486) -> (11.1453, 46.6377)
  line L556 (11.1453, 46.6377) -> (11.3158, 46.5958)
  line L557 (11.3158, 46.5958) -> (11.9247, 46.4436)
  line L558 (11.9247, 46.4436) -> (12.5316, 46.2837)
  line L559 (12.5316, 46.2837) -> (12.7012, 46.2382)
  line L560 (12.7012, 46.2382) -> (12.7234, 46.2385)
  line L561 (12.7234, 46.2385) -> (12.7718, 46.2557)
  line L562 (12.7718, 46.2557) -> (12.8246, 46.2953)
  line L563 (12.8246, 46.2953) -> (12.8809, 46.3575)
  line L564 (12.8809, 46.3575) -> (12.9398, 46.4424)
  line L565 (12.9398, 46.4424) -> (13.1561, 46.819)
  line L566 (13.1561, 46.819) -> (13.4548, 47.2993)
  line L567 (13.4548, 47.2993) -> (13.6295, 47.5617)
  line L568 (13.6295, 47.5617) -> (13.8205, 47.836)
  line L569 (13.8205, 47.836) -> (14.0303, 48.1242)
  line L570 (14.0303, 48.1242) -> (14.2584, 48.4241)
  line L571 (14.2584, 48.4241) -> (14.5046, 48.7341)
  line L572 (14.5046, 48.7341) -> (14.771, 49.0554)
  line L573 (14.771, 49.0554) -> (15.0578, 49.3871)
  line L574 (15.0578, 49.3871) -> (15.3297, 49.689)
  arc A16 (16.8045, 49.2098) -> (15.3297, 49.689) centre (0, 0) ccw
  line L575 (16.8045, 49.2098) -> (16.847, 48.8057)
  line L576 (16.847, 48.8057) -> (16.8841, 48.3688)
  line L577 (16.8841, 48.3688) -> (16.9107, 47.9523)
  line L578 (16.9107, 47.9523) -> (16.9277, 47.5567)
  line L579 (16.9277, 47.5567) -> (16.9359, 47.18)
  line L580 (16.9359, 47.18) -> (16.9363, 46.8236)
  line L581 (16.9363, 46.8236) -> (16.9296, 46.4894)
  line L582 (16.9296, 46.4894) -> (16.9167, 46.1745)
  line L583 (16.9167, 46.1745) -> (16.876, 45.6104)
  line L584 (16.876, 45.6104) -> (16.8297, 45.1785)
  line L585 (16.8297, 45.1785) -> (16.8273, 45.0752)
  line L586 (16.8273, 45.0752) -> (16.8363, 44.9918)
  line L587 (16.8363, 44.9918) -> (16.8558, 44.9287)
  line L588 (16.8558, 44.9287) -> (16.8848, 44.8864)
  line L589 (16.8848, 44.8864) -> (16.9027, 44.8731)
  line L590 (16.9027, 44.8731) -> (17.0666, 44.8102)
  line L591 (17.0666, 44.8102) -> (17.6516, 44.5828)
  line L592 (17.6516, 44.5828) -> (18.2337, 44.3481)
  line L593 (18.2337, 44.3481) -> (18.3962, 44.2817)
  line L594 (18.3962, 44.2817) -> (18.4183, 44.2792)
  line L595 (18.4183, 44.2792) -> (18.4685, 44.2902)
  line L596 (18.4685, 44.2902) -> (18.5258, 44.3229)
  line L597 (18.5258, 44.3229) -> (18.5895, 44.3775)
  line L598 (18.5895, 44.3775) -> (18.6585, 44.4544)
  line L599 (18.6585, 44.4544) -> (18.9203, 44.801)
  line L600 (18.9203, 44.801) -> (19.2769, 45.24)
  line L601 (19.2769, 45.24) -> (19.4831, 45.4785)
  line L602 (19.4831, 45.4785) -> (19.7069, 45.7266)
  line L603 (19.7069, 45.7266) -> (19.9512, 45.9862)
  line L604 (19.9512, 45.9862) -> (20.2151, 46.2552)
  line L605 (20.2151, 46.2552) -> (20.4983, 46.5319)
  line L606 (20.4983, 46.5319) -> (20.8028, 46.8173)
  line L607 (20.8028, 46.8173) -> (21.1289, 47.1104)
  line L608 (21.1289, 47.1104) -> (21.4365, 47.3759)
  arc A17 (22.8396, 46.7156) -> (21.4365, 47.3759) centre (0, 0) ccw
  line L609 (22.8396, 46.7156) -> (22.8311, 46.3094)
  line L610 (22.8311, 46.3094) -> (22.8132, 45.8713)
  line L611 (22.8132, 45.8713) -> (22.7874, 45.4547)
  line L612 (22.7874, 45.4547) -> (22.7546, 45.0601)
  line L613 (22.7546, 45.0601) -> (22.7156, 44.6854)
  line L614 (22.7156, 44.6854) -> (22.6713, 44.3317)
  line L615 (22.6713, 44.3317) -> (22.6228, 44.001)
  line L616 (22.6228, 44.001) -> (22.5705, 43.6902)
  line L617 (22.5705, 43.6902) -> (22.4595, 43.1356)
  line L618 (22.4595, 43.1356) -> (22.3593, 42.713)
  line L619 (22.3593, 42.713) -> (22.3441, 42.6107)
  line L620 (22.3441, 42.6107) -> (22.3425, 42.5269)
  line L621 (22.3425, 42.5269) -> (22.3539, 42.4618)
  line L622 (22.3539, 42.4618) -> (22.3774, 42.4162)
  line L623 (22.3774, 42.4162) -> (22.3935, 42.4008)
  line L624 (22.3935, 42.4008) -> (22.5482, 42.3178)
  line L625 (22.5482, 42.3178) -> (23.1001, 42.0189)
  line L626 (23.1001, 42.0189) -> (23.6482, 41.7131)
  line L627 (23.6482, 41.7131) -> (23.8011, 41.6269)
  line L628 (23.8011, 41.6269) -> (23.8227, 41.6216)
  line L629 (23.8227, 41.6216) -> (23.8739, 41.6262)
  line L630 (23.8739, 41.6262) -> (23.9349, 41.6515)
  line L631 (23.9349, 41.6515) -> (24.0049, 41.6977)
  line L632 (24.0049, 41.6977) -> (24.083, 41.7654)
  line L633 (24.083, 41.7654) -> (24.3862, 42.0763)
  line L634 (24.3862, 42.0763) -> (24.7949, 42.4673)
  line L635 (24.7949, 42.4673) -> (25.0294, 42.678)
  line L636 (25.0294, 42.678) -> (25.2826, 42.8961)
  line L637 (25.2826, 42.8961) -> (25.5575, 43.1231)
  line L638 (25.5575, 43.1231) -> (25.853, 43.3568)
  line L639 (25.853, 43.3568) -> (26.1686, 43.5959)
  line L640 (26.1686, 43.5959) -> (26.5065, 43.8409)
  line L641 (26.5065, 43.8409) -> (26.8668, 44.0908)
  line L642 (26.8668, 44.0908) -> (27.2052, 44.3156)
  arc A18 (28.5145, 43.4847) -> (27.2052, 44.3156) centre (0, 0) ccw
  line L643 (28.5145, 43.4847) -> (28.4552, 43.0827)
  line L644 (28.4552, 43.0827) -> (28.3825, 42.6503)
  line L645 (28.3825, 42.6503) -> (28.3047, 42.2403)
  line L646 (28.3047, 42.2403) -> (28.2227, 41.8529)
  line L647 (28.2227, 41.8529) -> (28.1371, 41.486)
  line L648 (28.1371, 41.486) -> (28.0488, 41.1407)
  line L649 (28.0488, 41.1407) -> (27.9592, 40.8187)
  line L650 (27.9592, 40.8187) -> (27.8684, 40.5168)
  line L651 (27.8684, 40.5168) -> (27.6887, 39.9805)
  line L652 (27.6887, 39.9805) -> (27.5364, 39.5738)
  line L653 (27.5364, 39.5738) -> (27.5084, 39.4743)
  line L654 (27.5084, 39.4743) -> (27.4964, 39.3913)
  line L655 (27.4964, 39.3913) -> (27.4995, 39.3253)
  line L656 (27.4995, 39.3253) -> (27.5171, 39.2771)
  line L657 (27.5171, 39.2771) -> (27.5311, 39.2598)
  line L658 (27.5311, 39.2598) -> (27.6742, 39.1581)
  line L659 (27.6742, 39.1581) -> (28.1843, 38.7924)
  line L660 (28.1843, 38.7924) -> (28.6898, 38.4203)
  line L661 (28.6898, 38.4203) -> (28.8307, 38.3156)
  line L662 (28.8307, 38.3156) -> (28.8515, 38.3076)
  line L663 (28.8515, 38.3076) -> (28.9028, 38.3058)
  line L664 (28.9028, 38.3058) -> (28.9665, 38.3232)
  line L665 (28.9665, 38.3232) -> (29.0417, 38.3603)
  line L666 (29.0417, 38.3603) -> (29.1277, 38.4176)
  line L667 (29.1277, 38.4176) -> (29.4675, 38.6882)
  line L668 (29.4675, 38.6882) -> (29.922, 39.0248)
  line L669 (29.922, 39.0248) -> (30.181, 39.2044)
  line L670 (30.181, 39.2044) -> (30.4596, 39.3891)
  line L671 (30.4596, 39.3891) -> (30.7607, 39.5798)
  line L672 (30.7607, 39.5798) -> (31.0832, 39.7747)
  line L673 (31.0832, 39.7747) -> (31.4263, 39.9723)
  line L674 (31.4263, 39.9723) -> (31.7922, 40.173)
  line L675 (31.7922, 40.173) -> (32.1809, 40.3758)
  line L676 (32.1809, 40.3758) -> (32.5449, 40.5565)
  arc A19 (33.7398, 39.568) -> (32.5449, 40.5565) centre (0, 0) ccw
  line L677 (33.7398, 39.568) -> (33.6305, 39.1766)
  line L678 (33.6305, 39.1766) -> (33.5042, 38.7568)
  line L679 (33.5042, 38.7568) -> (33.3756, 38.3597)
  line L680 (33.3756, 38.3597) -> (33.2458, 37.9857)
  line L681 (33.2458, 37.9857) -> (33.1148, 37.6324)
  line L682 (33.1148, 37.6324) -> (32.9839, 37.3008)
  line L683 (32.9839, 37.3008) -> (32.8546, 36.9926)
  line L684 (32.8546, 36.9926) -> (32.7267, 36.7045)
  line L685 (32.7267, 36.7045) -> (32.4812, 36.1949)
  line L686 (32.4812, 36.1949) -> (32.2791, 35.8105)
  line L687 (32.2791, 35.8105) -> (32.239, 35.7153)
  line L688 (32.239, 35.7153) -> (32.2166, 35.6344)
  line L689 (32.2166, 35.6344) -> (32.2115, 35.5686)
  line L690 (32.2115, 35.5686) -> (32.2229, 35.5186)
  line L691 (32.2229, 35.5186) -> (32.2346, 35.4996)
  line L692 (32.2346, 35.4996) -> (32.3638, 35.3808)
  line L693 (32.3638, 35.3808) -> (32.824, 34.954)
  line L694 (32.824, 34.954) -> (33.2789, 34.5215)
  line L695 (33.2789, 34.5215) -> (33.4056, 34.4)
  line L696 (33.4056, 34.4) -> (33.4252, 34.3895)
  line L697 (33.4252, 34.3895) -> (33.4759, 34.3813)
  line L698 (33.4759, 34.3813) -> (33.5412, 34.3905)
  line L699 (33.5412, 34.3905) -> (33.6205, 34.4179)
  line L700 (33.6205, 34.4179) -> (33.713, 34.464)
  line L701 (33.713, 34.464) -> (34.084, 34.6898)
  line L702 (34.084, 34.6898) -> (34.5771, 34.9668)
  line L703 (34.5771, 34.9668) -> (34.8566, 35.1126)
  line L704 (34.8566, 35.1126) -> (35.1561, 35.2609)
  line L705 (35.1561, 35.2609) -> (35.4788, 35.4124)
  line L706 (35.4788, 35.4124) -> (35.8232, 35.5653)
  line L707 (35.8232, 35.5653) -> (36.1883, 35.7184)
  line L708 (36.1883, 35.7184) -> (36.5765, 35.8717)
  line L709 (36.5765, 35.8717) -> (36.9876, 36.0241)
  line L710 (36.9876, 36.0241) -> (37.3714, 36.1577)
  arc A20 (38.4329, 35.0273) -> (37.3714, 36.1577) centre (0, 0) ccw
  line L711 (38.4329, 35.0273) -> (38.2755, 34.6527)
  line L712 (38.2755, 34.6527) -> (38.0975, 34.252)
  line L713 (38.0975, 34.252) -> (37.9202, 33.8742)
  line L714 (37.9202, 33.8742) -> (37.7445, 33.5193)
  line L715 (37.7445, 33.5193) -> (37.5702, 33.1852)
  line L716 (37.5702, 33.1852) -> (37.3988, 32.8727)
  line L717 (37.3988, 32.8727) -> (37.232, 32.5831)
  line L718 (37.232, 32.5831) -> (37.069, 32.3133)
  line L719 (37.069, 32.3133) -> (36.7615, 31.8386)
  line L720 (36.7615, 31.8386) -> (36.5129, 31.4825)
  line L721 (36.5129, 31.4825) -> (36.4611, 31.3931)
  line L722 (36.4611, 31.3931) -> (36.4288, 31.3156)
  line L723 (36.4288, 31.3156) -> (36.4154, 31.251)
  line L724 (36.4154, 31.251) -> (36.4205, 31.1999)
  line L725 (36.4205, 31.1999) -> (36.4297, 31.1796)
  line L726 (36.4297, 31.1796) -> (36.543, 31.0456)
  line L727 (36.543, 31.0456) -> (36.9461, 30.5645)
  line L728 (36.9461, 30.5645) -> (37.3431, 30.0784)
  line L729 (37.3431, 30.0784) -> (37.4536, 29.942)
  line L730 (37.4536, 29.942) -> (37.4718, 29.9291)
  line L731 (37.4718, 29.9291) -> (37.521, 29.9145)
  line L732 (37.521, 29.9145) -> (37.587, 29.9155)
  line L733 (37.587, 29.9155) -> (37.6691, 29.9328)
  line L734 (37.6691, 29.9328) -> (37.7667, 29.9669)
  line L735 (37.7667, 29.9669) -> (38.163, 30.1444)
  line L736 (38.163, 30.1444) -> (38.687, 30.3574)
  line L737 (38.687, 30.3574) -> (38.9826, 30.467)
  line L738 (38.9826, 30.467) -> (39.2983, 30.5766)
  line L739 (39.2983, 30.5766) -> (39.6374, 30.6865)
  line L740 (39.6374, 30.6865) -> (39.9982, 30.795)
  line L741 (39.9982, 30.795) -> (40.3797, 30.9011)
  line L742 (40.3797, 30.9011) -> (40.784, 31.0045)
  line L743 (40.784, 31.0045) -> (41.211, 31.1042)
  line L744 (41.211, 31.1042) -> (41.6085, 31.1887)
  arc A21 (42.5199, 29.9342) -> (41.6085, 31.1887) centre (0, 0) ccw
  line L745 (42.5199, 29.9342) -> (42.3168, 29.5822)
  line L746 (42.3168, 29.5822) -> (42.09, 29.207)
  line L747 (42.09, 29.207) -> (41.8667, 28.8544)
  line L748 (41.8667, 28.8544) -> (41.6479, 28.5244)
  line L749 (41.6479, 28.5244) -> (41.4332, 28.2148)
  line L750 (41.4332, 28.2148) -> (41.224, 27.9262)
  line L751 (41.224, 27.9262) -> (41.0221, 27.6598)
  line L752 (41.0221, 27.6598) -> (40.8266, 27.4126)
  line L753 (40.8266, 27.4126) -> (40.4621, 26.9801)
  line L754 (40.4621, 26.9801) -> (40.1708, 26.658)
  line L755 (40.1708, 26.658) -> (40.1081, 26.5757)
  line L756 (40.1081, 26.5757) -> (40.0664, 26.503)
  line L757 (40.0664, 26.503) -> (40.045, 26.4405)
  line L758 (40.045, 26.4405) -> (40.0436, 26.3892)
  line L759 (40.0436, 26.3892) -> (40.0503, 26.3679)
  line L760 (40.0503, 26.3679) -> (40.1459, 26.2207)
  line L761 (40.1459, 26.2207) -> (40.4855, 25.6929)
  line L762 (40.4855, 25.6929) -> (40.8185, 25.1609)
  line L763 (40.8185, 25.1609) -> (40.911, 25.0117)
  line L764 (40.911, 25.0117) -> (40.9274, 24.9966)
  line L765 (40.9274, 24.9966) -> (40.9744, 24.976)
  line L766 (40.9744, 24.976) -> (41.04, 24.9687)
  line L767 (41.04, 24.9687) -> (41.1237, 24.9755)
  line L768 (41.1237, 24.9755) -> (41.2247, 24.9972)
  line L769 (41.2247, 24.9972) -> (41.6402, 25.1237)
  line L770 (41.6402, 25.1237) -> (42.1867, 25.2693)
  line L771 (42.1867, 25.2693) -> (42.4937, 25.341)
  line L772 (42.4937, 25.341) -> (42.8207, 25.4102)
  line L773 (42.8207, 25.4102) -> (43.1709, 25.4766)
  line L774 (43.1709, 25.4766) -> (43.5425, 25.5391)
  line L775 (43.5425, 25.5391) -> (43.9342, 25.5966)
  line L776 (43.9342, 25.5966) -> (44.3483, 25.6485)
  line L777 (44.3483, 25.6485) -> (44.7844, 25.6939)
  line L778 (44.7844, 25.6939) -> (45.1894, 25.7278)
  arc A22 (45.9364, 24.369) -> (45.1894, 25.7278) centre (0, 0) ccw
  line L779 (45.9364, 24.369) -> (45.6907, 24.0453)
  line L780 (45.6907, 24.0453) -> (45.4187, 23.7014)
  line L781 (45.4187, 23.7014) -> (45.153, 23.3796)
  line L782 (45.153, 23.3796) -> (44.8946, 23.0796)
  line L783 (44.8946, 23.0796) -> (44.6427, 22.7993)
  line L784 (44.6427, 22.7993) -> (44.399, 22.5393)
  line L785 (44.399, 22.5393) -> (44.1654, 22.3002)
  line L786 (44.1654, 22.3002) -> (43.9404, 22.0795)
  line L787 (43.9404, 22.0795) -> (43.5245, 21.6961)
  line L788 (43.5245, 21.6961) -> (43.1951, 21.413)
  line L789 (43.1951, 21.413) -> (43.1227, 21.3393)
  line L790 (43.1227, 21.3393) -> (43.0722, 21.2723)
  line L791 (43.0722, 21.2723) -> (43.0431, 21.213)
  line L792 (43.0431, 21.213) -> (43.0353, 21.1623)
  line L793 (43.0353, 21.1623) -> (43.0393, 21.1404)
  line L794 (43.0393, 21.1404) -> (43.1157, 20.9823)
  line L795 (43.1157, 20.9823) -> (43.3865, 20.4161)
  line L796 (43.3865, 20.4161) -> (43.6501, 19.8465)
  line L797 (43.6501, 19.8465) -> (43.7232, 19.6869)
  line L798 (43.7232, 19.6869) -> (43.7376, 19.6699)
  line L799 (43.7376, 19.6699) -> (43.7817, 19.6436)
  line L800 (43.7817, 19.6436) -> (43.8458, 19.6282)
  line L801 (43.8458, 19.6282) -> (43.9297, 19.6244)
  line L802 (43.9297, 19.6244) -> (44.0326, 19.6332)
  line L803 (44.0326, 19.6332) -> (44.4607, 19.7066)
  line L804 (44.4607, 19.7066) -> (45.0212, 19.7826)
  line L805 (45.0212, 19.7826) -> (45.3347, 19.8153)
  line L806 (45.3347, 19.8153) -> (45.6678, 19.8429)
  line L807 (45.6678, 19.8429) -> (46.0235, 19.865)
  line L808 (46.0235, 19.865) -> (46.4, 19.8804)
  line L809 (46.4, 19.8804) -> (46.7959, 19.8883)
  line L810 (46.7959, 19.8883) -> (47.2132, 19.8879)
  line L811 (47.2132, 19.8879) -> (47.6516, 19.8783)
  line L812 (47.6516, 19.8783) -> (48.0576, 19.8612)
  arc A23 (48.6284, 18.4194) -> (48.0576, 19.8612) centre (0, 0) ccw
  line L813 (48.6284, 18.4194) -> (48.3441, 18.1291)
  line L814 (48.3441, 18.1291) -> (48.0312, 17.822)
  line L815 (48.0312, 17.822) -> (47.7272, 17.536)
  line L816 (47.7272, 17.536) -> (47.4332, 17.2708)
  line L817 (47.4332, 17.2708) -> (47.1482, 17.0243)
  line L818 (47.1482, 17.0243) -> (46.8738, 16.7969)
  line L819 (46.8738, 16.7969) -> (46.6121, 16.589)
  line L820 (46.6121, 16.589) -> (46.3612, 16.3982)
  line L821 (46.3612, 16.3982) -> (45.9006, 16.0699)
  line L822 (45.9006, 16.0699) -> (45.5383, 15.8304)
  line L823 (45.5383, 15.8304) -> (45.4572, 15.7663)
  line L824 (45.4572, 15.7663) -> (45.3987, 15.7062)
  line L825 (45.3987, 15.7062) -> (45.3624, 15.651)
  line L826 (45.3624, 15.651) -> (45.3483, 15.6017)
  line L827 (45.3483, 15.6017) -> (45.3495, 15.5794)
  line L828 (45.3495, 15.5794) -> (45.4055, 15.4131)
  line L829 (45.4055, 15.4131) -> (45.6032, 14.8174)
  line L830 (45.6032, 14.8174) -> (45.7934, 14.2192)
  line L831 (45.7934, 14.2192) -> (45.8459, 14.0517)
  line L832 (45.8459, 14.0517) -> (45.858, 14.0331)
  line L833 (45.858, 14.0331) -> (45.8984, 14.0014)
  line L834 (45.8984, 14.0014) -> (45.9602, 13.9781)
  line L835 (45.9602, 13.9781) -> (46.0429, 13.9638)
  line L836 (46.0429, 13.9638) -> (46.1461, 13.9597)
  line L837 (46.1461, 13.9597) -> (46.58, 13.9788)
  line L838 (46.58, 13.9788) -> (47.1456, 13.984)
  line L839 (47.1456, 13.984) -> (47.4607, 13.9771)
  line L840 (47.4607, 13.9771) -> (47.7946, 13.9628)
  line L841 (47.7946, 13.9628) -> (48.1504, 13.9401)
  line L842 (48.1504, 13.9401) -> (48.5258, 13.9082)
  line L843 (48.5258, 13.9082) -> (48.9196, 13.8664)
  line L844 (48.9196, 13.8664) -> (49.3336, 13.8137)
  line L845 (49.3336, 13.8137) -> (49.7672, 13.7492)
  line L846 (49.7672, 13.7492) -> (50.1679, 13.6814)
  arc A24 (50.5535, 12.1794) -> (50.1679, 13.6814) centre (0, 0) ccw
  line L847 (50.5535, 12.1794) -> (50.2351, 11.927)
  line L848 (50.2351, 11.927) -> (49.8861, 11.6616)
  line L849 (49.8861, 11.6616) -> (49.5487, 11.416)
  line L850 (49.5487, 11.416) -> (49.2238, 11.1897)
  line L851 (49.2238, 11.1897) -> (48.9102, 10.9808)
  line L852 (48.9102, 10.9808) -> (48.6094, 10.7896)
  line L853 (48.6094, 10.7896) -> (48.3237, 10.6162)
  line L854 (48.3237, 10.6162) -> (48.0508, 10.4583)
  line L855 (48.0508, 10.4583) -> (47.5527, 10.1903)
  line L856 (47.5527, 10.1903) -> (47.1633, 9.9981)
  line L857 (47.1633, 9.9981) -> (47.0748, 9.9447)
  line L858 (47.0748, 9.9447) -> (47.0092, 9.8924)
  line L859 (47.0092, 9.8924) -> (46.9663, 9.8422)
  line L860 (46.9663, 9.8422) -> (46.9461, 9.795)
  line L861 (46.9461, 9.795) -> (46.9445, 9.7728)
  line L862 (46.9445, 9.7728) -> (46.9792, 9.6007)
  line L863 (46.9792, 9.6007) -> (47.1007, 8.9849)
  line L864 (47.1007, 8.9849) -> (47.2144, 8.3677)
  line L865 (47.2144, 8.3677) -> (47.2455, 8.1949)
  line L866 (47.2455, 8.1949) -> (47.2552, 8.1749)
  line L867 (47.2552, 8.1749) -> (47.2914, 8.1384)
  line L868 (47.2914, 8.1384) -> (47.3497, 8.1075)
  line L869 (47.3497, 8.1075) -> (47.4299, 8.083)
  line L870 (47.4299, 8.083) -> (47.5319, 8.0659)
  line L871 (47.5319, 8.0659) -> (47.9647, 8.0306)
  line L872 (47.9647, 8.0306) -> (48.5265, 7.9648)
  line L873 (48.5265, 7.9648) -> (48.8383, 7.9185)
  line L874 (48.8383, 7.9185) -> (49.1678, 7.8624)
  line L875 (49.1678, 7.8624) -> (49.5178, 7.7953)
  line L876 (49.5178, 7.7953) -> (49.8863, 7.7166)
  line L877 (49.8863, 7.7166) -> (50.2717, 7.6258)
  line L878 (50.2717, 7.6258) -> (50.6759, 7.5216)
  line L879 (50.6759, 7.5216) -> (51.098, 7.4033)
  line L880 (51.098, 7.4033) -> (51.487, 7.2858)
  arc A25 (51.6814, 5.7474) -> (51.487, 7.2858) centre (0, 0) ccw
  line L881 (51.6814, 5.7474) -> (51.3338, 5.5368)
  line L882 (0, 6.6742) -> (0, 47.95)
  line L883 (6.6666, -0.3178) -> (47.8961, -2.2835)
  arc A26 (0, 6.6742) -> (6.6666, -0.3178) centre (7, 6.6742) ccw
  point P0 (0, 0)
  point P1 (51.9942, -0.7753)
  point P2 (51.9942, 0.7753)
  point P3 (51.6814, 5.7474)
  point P4 (51.487, 7.2858)
  point P5 (50.5535, 12.1794)
  point P6 (50.1679, 13.6814)
  point P7 (48.6284, 18.4194)
  point P8 (48.0576, 19.8612)
  point P9 (45.9364, 24.369)
  point P10 (45.1894, 25.7278)
  point P11 (42.5199, 29.9342)
  point P12 (41.6085, 31.1887)
  point P13 (38.4329, 35.0273)
  point P14 (37.3714, 36.1577)
  point P15 (33.7398, 39.568)
  point P16 (32.5449, 40.5565)
  point P17 (28.5145, 43.4847)
  point P18 (27.2052, 44.3156)
  point P19 (22.8396, 46.7156)
  point P20 (21.4365, 47.3759)
  point P21 (16.8045, 49.2098)
  point P22 (15.3297, 49.689)
  point P23 (10.5044, 50.928)
  point P24 (8.9811, 51.2185)
  point P25 (4.0386, 51.8429)
  point P26 (2.4909, 51.9403)
  dimension "d0" = 7
  constraints: 1768 end point, 54 point on circle, 27 centre point, 2 point on line, 2 tangent, 1 vertical
  measures "d0" radius of A26
extrude "Extrusion1" add sketch "Sketch1" along normal blind 7
sketch "Sketch2" plane through (0, 0, 0) normal (-1, 0, 0) x (0, 0, 1)
  circle A0 centre (6.6742, 7) radius 2.475
  arc A1 (-0.3178, 6.6666) -> (6.6742, 0) centre (6.6742, 7) ccw projected
  point P0 (0, 0)
  dimension "d3" = 4.95
  constraints: 1 centre point, 1 concentric
  measures "d3" diameter of A0
extrude "Extrusion2" add sketch "Sketch2" along normal blind 8.1
chamfer "Chamfer1" distance 0.5 angle 45 1 edges at (-8.1, 7, 4.1992)